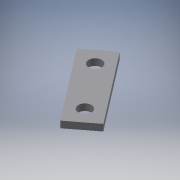
# Autodesk Inventor part: gantry_y_holder
Saved by Autodesk Inventor 2016 SP2 (Build 200236200, 236)
## iProperties
Created: 2017-09-10
Part Number: gantry_y_holder
Material: Generic
Document SubType Name: Modeling
Designer: Admin
Density: 1 g/cm^3
Appearance: Default
Author: Admin
Autodesk Inventor part; units mm, degrees
ref_plane "YZ Plane" through (0, 0, 0) normal (1, 0, 0) x (0, 1, 0)
ref_plane "XZ Plane" through (0, 0, 0) normal (0, 1, 0) x (-1, 0, 0)
ref_plane "XY Plane" through (0, 0, 0) normal (0, 0, 1) x (1, 0, 0)
sketch "Sketch1" plane through (0, 0, 0) normal (0, 0, 1) x (1, 0, 0)
  circle A0 centre (0, 0) radius 15 projected
  circle A1 centre (77.2853, -100.6476) radius 15 projected
  line L0 (0, 0) -> (77.2853, -100.6476) construction
  line L1 (4.6165, 51.4557) -> (140.1218, -125.0109) construction
  line L2 (-50.9034, 8.823) -> (49.7593, -122.2685) construction
  line L3 (11.1166, -71.9447) -> (66.6365, -29.312) construction
  line L4 (-50.9034, 8.823) -> (4.6165, 51.4557) construction
  line L5 (82.3144, -169.4001) -> (140.1218, -125.0109) construction
  line L6 (-50.9034, 8.823) -> (4.6165, 51.4557)
  line L7 (4.6165, 51.4557) -> (128.1887, -109.4706)
  line L8 (128.1887, -109.4706) -> (72.6688, -152.1033)
  line L9 (72.6688, -152.1033) -> (-50.9034, 8.823)
  point P0 (0, 0)
  dimension "d0" = 38
  dimension "d1" = 38
  dimension "d2" = 35
  dimension "d3" = 35
  constraints: 20 end point, 6 parallel, 2 point on line, 1 collinear, 1 perpendicular
  measures "d0" distance from line of L4 point (0, 0)
  measures "d1" distance from line of L8 L0.end
  measures "d2" distance from line of L1 point (0, 0)
  measures "d3" distance from line of L2 point (0, 0)
extrude "Extrusion1" add sketch "Sketch1" along normal blind 15
body "Solid1"
